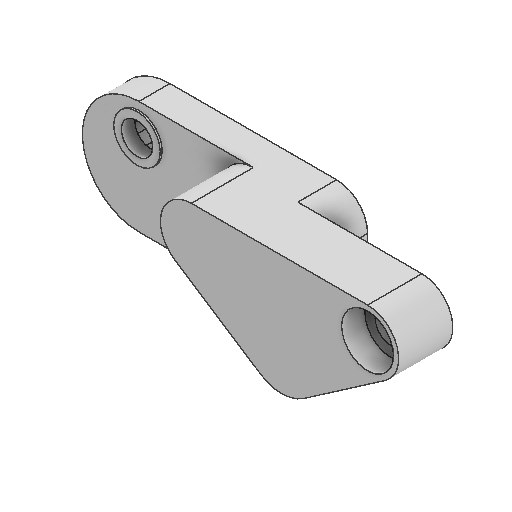
# Autodesk Inventor part: b link
Saved by Autodesk Inventor 2025 (Build 290162000, 162)
## iProperties
Created: 2025-01-09
Part Number: b link
Material: Generic
Document SubType Name: Modeling
Designer: derm
Density: 1 g/cm^3
Appearance: Default
Author: derm
Autodesk Inventor part; units mm, degrees
ref_plane "YZ Plane" through (0, 0, 0) normal (1, 0, 0) x (0, 1, 0)
ref_plane "XZ Plane" through (0, 0, 0) normal (0, 1, 0) x (-1, 0, 0)
ref_plane "XY Plane" through (0, 0, 0) normal (0, 0, 1) x (1, 0, 0)
sketch "Sketch1" plane through (0, 0, 0) normal (0, 0, 1) x (1, 0, 0)
  line L0 (0, 0) -> (75, 0) construction
  line L1 (0, -8) -> (75, -8)
  line L2 (75, 8) -> (0, 8)
  arc A0 (0, 8) -> (0, -8) centre (0, 0) ccw
  arc A1 (75, -8) -> (75, 8) centre (75, 0) ccw
  circle A2 centre (0, 0) radius 4.05
  circle A3 centre (75, 0) radius 4.05
  point P0 (37.5, 0)
  dimension "d0" = 75
  dimension "d1" = 8
  dimension "d2" = 8.1
  constraints: 8 end point, 4 centre point, 4 point on circle, 4 tangent, 2 coincident, 1 equal radius, 1 horizontal, 1 midpoint, 1 parallel
  measures "d0" distance of L0.start L0.end
  measures "d1" radius of A0
  measures "d2" diameter of A3
extrude "Extrusion1" add sketch "Sketch1" along normal blind 10
sketch "Sketch2" plane through (0, 0, 0) normal (0, 0, -1) x (-1, 0, 0)
  arc A0 (-75, 8) -> (-75, -8) centre (-75, 0) ccw projected
  line L0 (0, -8) -> (-75, -8) projected
  arc A1 (0, -8) -> (0, 8) centre (0, 0) ccw projected
  line L1 (-75, 8) -> (0, 8) projected
  circle A2 centre (-75, 0) radius 4.05 projected
  circle A3 centre (0, 0) radius 4.05 projected
  line L2 (0, 0) -> (-43.0059, 0) construction
  line L3 (0, -8) -> (-43.0059, -8)
  line L4 (-43.0059, 8) -> (0, 8)
  arc A4 (0, -8) -> (0, 8) centre (0, 0) ccw
  arc A5 (-43.0059, 8) -> (-43.0059, -8) centre (-43.0059, 0) ccw
  point P0 (-21.503, 0)
  constraints: 8 end point, 4 point on circle, 4 tangent, 2 centre point, 1 horizontal, 1 midpoint, 1 parallel
extrude "Extrusion2" add sketch "Sketch2" along normal blind 10 contours L1 A1 L0 A5
sketch "Sketch3" plane through (0, 0, 10) normal (0, 0, 1) x (1, 0, 0)
  arc A0 (75, -8) -> (75, 8) centre (75, 0) ccw projected
  line L0 (75, 8) -> (0, 8) projected
  arc A1 (0, 8) -> (0, -8) centre (0, 0) ccw projected
  line L1 (0, -8) -> (75, -8) projected
  circle A2 centre (75, 0) radius 4.05 projected
  circle A3 centre (0, 0) radius 4.05 projected
  line L2 (75, 0) -> (29.5329, 0) construction
  line L3 (75, -8) -> (29.5329, -8)
  line L4 (29.5329, 8) -> (75, 8)
  arc A4 (75, -8) -> (75, 8) centre (75, 0) ccw
  arc A5 (29.5329, 8) -> (29.5329, -8) centre (29.5329, 0) ccw
  point P0 (52.2664, 0)
  constraints: 8 end point, 4 point on circle, 4 tangent, 2 centre point, 1 horizontal, 1 midpoint, 1 parallel
extrude "Extrusion3" cut sketch "Sketch3" against normal blind 10 contours L1 A1 L0 A5
sketch "Sketch4" plane through (0, 0, 10) normal (0, 0, 1) x (1, 0, 0)
  circle A0 centre (75, 0) radius 4.05 projected
  arc A1 (29.5329, 8) -> (29.5329, -8) centre (29.5329, 0) ccw projected
  line L0 (29.5329, -8) -> (75, -8) projected
  arc A2 (75, -8) -> (75, 8) centre (75, 0) ccw projected
  line L1 (75, 8) -> (29.5329, 8) projected
  line L2 (25.1547, -6.6956) -> (53.0225, -24.918)
  line L3 (53.0225, -24.918) -> (79.5491, -6.5807)
  arc A3 (75, -8) -> (75, 8) centre (75, 0) ccw projected
  point P0 (0, 0)
  point P1 (79.5491, -6.5807)
  constraints: 4 end point, 2 point on circle, 2 tangent
extrude "Extrusion4" add sketch "Sketch4" against normal blind 10 contours A1 L0 A2 L3 L2
fillet "Fillet1" radius 10 1 edges at (53.0225, -24.918, 5)
sketch "Sketch5" plane through (0, 0, 0) normal (0, 0, 1) x (1, 0, 0)
  line L0 (27.1495, -8) -> (25.1547, -6.6956) projected
  arc A0 (29.5329, 8) -> (25.1547, -6.6956) centre (29.5329, 0) ccw projected
  line L1 (0, 8) -> (29.5329, 8) projected
  arc A1 (0, 8) -> (0, -8) centre (0, 0) ccw projected
  line L2 (27.1495, -8) -> (0, -8) projected
  circle A2 centre (0, 0) radius 4.05 projected
extrude "Extrusion5" cut sketch "Sketch5" against normal blind 2
sketch "Sketch6" plane through (0, 0, -10) normal (0, 0, -1) x (-1, 0, 0)
  circle A0 centre (0, 0) radius 4.05 projected
  arc A1 (0, -8) -> (0, 8) centre (0, 0) ccw projected
  circle A2 centre (0, 0) radius 6.581
  constraints: 1 centre point, 1 coincident
extrude "Extrusion6" cut sketch "Sketch6" against normal blind 5
sketch "Sketch7" plane through (0, 0, -2) normal (0, 0, 1) x (1, 0, 0)
  line L0 (27.1495, -8) -> (0, -8) projected
  line L1 (25.1547, -6.6956) -> (27.1495, -8) projected
  arc A0 (29.5329, 8) -> (25.1547, -6.6956) centre (29.5329, 0) ccw projected
  line L2 (0, 8) -> (29.5329, 8) projected
  arc A1 (0, 8) -> (0, -8) centre (0, 0) ccw projected
  circle A2 centre (0, 0) radius 4.05 projected
  circle A3 centre (0, 0) radius 6.0105
  constraints: 1 centre point, 1 coincident
extrude "Extrusion7" add sketch "Sketch7" along normal blind 0.5 contours A3
sketch "Sketch8" plane through (0, 0, 0) normal (0, 0, -1) x (-1, 0, 0)
  arc A0 (-58.5537, -21.0944) -> (-47.3946, -21.238) centre (-52.8674, -12.8685) ccw projected
  line L0 (-47.3946, -21.238) -> (-27.1495, -8) projected
  line L1 (-43.0059, -8) -> (-27.1495, -8) projected
  arc A1 (-43.0059, 8) -> (-43.0059, -8) centre (-43.0059, 0) ccw projected
  line L2 (-75, 8) -> (-43.0059, 8) projected
  arc A2 (-75, 8) -> (-79.5491, -6.5807) centre (-75, 0) ccw projected
  line L3 (-79.5491, -6.5807) -> (-58.5537, -21.0944) projected
  circle A3 centre (-75, 0) radius 4.05 projected
  circle A4 centre (-75, 0) radius 7.0719
  point P0 (0, 0)
  constraints: 1 centre point, 1 coincident
extrude "Extrusion8" add sketch "Sketch8" along normal blind 0.5 contours A4
sketch "Sketch9" plane through (0, 0, -10) normal (0, 0, -1) x (-1, 0, 0)
  circle A0 centre (0, 0) radius 6.581 projected
  line L0 (-43.0059, -8) -> (0, -8) projected
  arc A1 (0, -8) -> (0, 8) centre (0, 0) ccw projected
  line L1 (0, 8) -> (-43.0059, 8) projected
  arc A2 (-43.0059, 8) -> (-43.0059, -8) centre (-43.0059, 0) ccw projected
  line L2 (0, -6.581) -> (-36.425, -6.581) construction
  line L3 (0, 8) -> (-36.425, 8)
  line L4 (-36.425, -21.1619) -> (0, -21.1619)
  arc A3 (0, -21.1619) -> (0, 8) centre (0, -6.581) ccw
  arc A4 (-36.425, 8) -> (-36.425, -21.1619) centre (-36.425, -6.581) ccw
  line L5 (0, 8) -> (-43.0059, 8) projected
  arc A5 (0, -8) -> (0, 8) centre (0, 0) ccw projected
  line L6 (-51.0059, -6.581) -> (-51.0059, 0)
  point P0 (-18.2125, -6.581)
  point P1 (0, 8)
  point P2 (-50.5041, -2.7887)
  constraints: 10 end point, 6 point on circle, 6 tangent, 2 centre point, 2 parallel, 1 collinear, 1 horizontal, 1 midpoint, 1 vertical, 1 vertical alignment, 1 other
extrude "Extrusion9" add sketch "Sketch9" against normal up to surface (8 mm away) contours L0 A1 A3 L4 A4 A2 | A4 L6 A2
sketch "Sketch10" plane through (0, 0, -2) normal (0, 0, 1) x (1, 0, 0)
  arc A0 (47.3946, -21.238) -> (58.5537, -21.0944) centre (52.8674, -12.8685) ccw projected
  line L0 (58.5537, -21.0944) -> (79.5491, -6.5807) projected
  arc A1 (79.5491, -6.5807) -> (75, 8) centre (75, 0) ccw projected
  line L1 (75, 8) -> (29.5329, 8) projected
  arc A2 (29.5329, 8) -> (25.1547, -6.6956) centre (29.5329, 0) ccw projected
  line L2 (25.1547, -6.6956) -> (47.3946, -21.238) projected
  circle A3 centre (75, 0) radius 4.05 projected
  circle A4 centre (0, 0) radius 6.0105 projected
  line L3 (25.1547, -6.6956) -> (27.1495, -8) projected
  arc A5 (29.5329, 8) -> (25.1547, -6.6956) centre (29.5329, 0) ccw projected
  line L4 (0, 8) -> (29.5329, 8) projected
  arc A6 (0, 8) -> (0, -21.1619) centre (0, -6.581) ccw projected
  line L5 (36.425, -21.1619) -> (0, -21.1619) projected
  arc A7 (36.425, -21.1619) -> (51.0059, -6.581) centre (36.425, -6.581) ccw projected
  line L6 (51.0059, 0) -> (51.0059, -6.581) projected
  arc A8 (43.0059, -8) -> (51.0059, 0) centre (43.0059, 0) ccw projected
  line L7 (27.1495, -8) -> (43.0059, -8) projected
  point P0 (44.017, -19.0294)
extrude "Extrusion10" add sketch "Sketch10" along normal up to surface (2 mm away) contours L2 L7 A8 L6 A7
sketch "Sketch11" plane through (0, 0, 10) normal (0, 0, 1) x (1, 0, 0)
  arc A0 (47.3946, -21.238) -> (58.5537, -21.0944) centre (52.8674, -12.8685) ccw projected
  line L0 (58.5537, -21.0944) -> (79.5491, -6.5807) projected
  arc A1 (79.5491, -6.5807) -> (75, 8) centre (75, 0) ccw projected
  line L1 (75, 8) -> (29.5329, 8) projected
  arc A2 (29.5329, 8) -> (25.1547, -6.6956) centre (29.5329, 0) ccw projected
  line L2 (25.1547, -6.6956) -> (47.3946, -21.238) projected
  circle A3 centre (75, 0) radius 4.05 projected
  circle A4 centre (75, 0) radius 6.6956
  point P0 (0, 0)
  constraints: 1 centre point, 1 coincident
extrude "Extrusion11" cut sketch "Sketch11" against normal blind 2 contours A4
thicken "Thicken1" operation add thickness 4 both sides no extend neighbours no toward (0, 0, 1) faces at (48.4106, -4.4127, 10)
sketch "Sketch12" plane through (0, 0, -10) normal (0, 0, -1) x (-1, 0, 0)
  circle A0 centre (0, 0) radius 4.05 projected
  line L0 (-7.5056, 0) -> (-3.7528, 6.5)
  line L1 (-3.7528, 6.5) -> (3.7528, 6.5)
  line L2 (3.7528, 6.5) -> (7.5056, 0)
  line L3 (7.5056, 0) -> (3.7528, -6.5)
  line L4 (3.7528, -6.5) -> (-3.7528, -6.5)
  line L5 (-3.7528, -6.5) -> (-7.5056, 0)
  dimension "d28" = 13
  constraints: 12 end point, 1 coincident, 13 other
  measures "d28" distance between parallel lines of L3 L0
extrude "Extrusion12" cut sketch "Sketch12" against normal up to surface (5 mm away)
body "Solid1"
